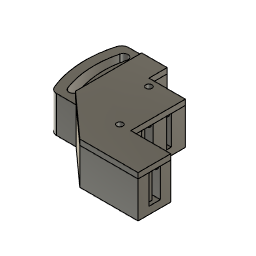
switch_connectors (Autodesk Fusion 360 design; units mm, degrees)
Autodesk Fusion 360 part; units mm, degrees
note: some values were not read from the file. Chosen so that the rebuilt part matches the saved one: which bodies a step acts on; which face or edge a step refers to. Set by a fixed rule: which sketch regions a step uses.
ref_plane "WorkPlane1" through (11.25, 0, 0) normal (1, 0, 0) x (0, 1, 0)
sketch "switch_connector" plane through (0, 0, 0) normal (0, 0, 1) x (1, 0, 0)
  line L0 (-55, 15) -> (-25, 15)
  line L1 (-25, 15) -> (-25, 0)
  line L2 (-25, 0) -> (-55, 0)
  line L3 (-55, 0) -> (-55, 15)
  line L4 (-44, -3) -> (-44, 0)
  line L5 (-43.2133, 0) -> (-43.2133, -4)
  line L6 (-43.2133, -4) -> (-55, -4)
  line L7 (-55, -4) -> (-55, -3)
  line L8 (-55, -3) -> (-44, -3)
  line L9 (-66, 5) -> (-55, 5)
  line L10 (-66, 5) -> (-66, 6)
  line L11 (-66, 6) -> (-55, 6)
  line L12 (-66, 10) -> (-66, 11)
  line L13 (-66, 11) -> (-55, 11)
  line L14 (-55, 10) -> (-66, 10)
  line L15 (-72, 15) -> (-44, 15)
  line L16 (-44, 15) -> (-44, -9)
  line L17 (-44, -9) -> (-72, -9)
  line L18 (-72, -9) -> (-72, 15)
  line L19 (-60, -9) -> (-72, 1.8)
  line L20 (-55, 3.5) -> (-66, 3.5)
  line L21 (-66, 3.5) -> (-66, 3)
  line L22 (-66, 3) -> (-55, 3)
  circle A0 centre (-61, 2.5) radius 1.0194
  line L23 (-63, -1.3962) -> (-60.2264, 1.8361)
  line L24 (-61.8884, 3) -> (-65, 1)
  line L25 (-65, -3) -> (-71, 3)
  line L26 (-71, 3) -> (-71, 15)
  line L27 (-65, 1) -> (-68, 4.3653)
  line L28 (-68, 4.3653) -> (-68, 15)
  line L29 (-56, 3.5) -> (-56, 5)
  line L30 (-44, -5.5) -> (-55, -5.5)
  line L31 (-55, -5.5) -> (-55, -6)
  line L32 (-55, -6) -> (-44, -6)
  line L33 (-44, -6) -> (-44, -5.5)
  line L34 (-45, -5.5) -> (-45, -4)
  circle A1 centre (-55.5, -6.5) radius 1.118
  line L35 (-63, -1.3962) -> (-55, -5.5)
  line L36 (-65, -3) -> (-58.0664, -7.5028)
  line L37 (-58.0664, -7.5028) -> (-55.5506, -7.6169)
  circle A2 centre (-58, 0) radius 0.65
  arc A3 (-75, 18) -> (-74.1574, 3.3947) centre (-52, 12) ccw
  circle A4 centre (-75, 18) radius 1.25
  circle A5 centre (-74.1574, 3.3947) radius 1.25
  line L38 (-74.0903, 17.5501) -> (-74.0625, 17.6607)
  arc A6 (-78.4578, 19.5487) -> (-77.3721, 1.3578) centre (-52, 12) ccw
  line L39 (-71, 15) -> (-71, 19)
  line L40 (-73, 21) -> (-76.5346, 21)
  line L41 (-75.5278, 0.1314) -> (-72, 0.1314)
  arc A7 (-71, 19) -> (-73, 21) centre (-73, 19) ccw
  arc A8 (-76.5346, 21) -> (-78.4578, 19.5487) centre (-76.5346, 19) ccw
  arc A9 (-77.3721, 1.3578) -> (-75.5278, 0.1314) centre (-75.5278, 2.1314) ccw
  arc A10 (-76.2263, 18.2423) -> (-75.3023, 2.896) centre (-52, 12) ccw
  arc A11 (-73.8338, 17.5501) -> (-73.0477, 3.9681) centre (-52, 12) ccw
  line L42 (-72, 12.1082) -> (-65, 12.1082)
  line L43 (-65, 12.1082) -> (-65, 20)
  line L44 (-65, 20) -> (-72, 20)
  line L45 (-72, 20) -> (-72, 12.1082)
  line L46 (-67, 20) -> (-67, 15)
  circle A12 centre (-63, 13) radius 0.65
  line L47 (-72, 0.1314) -> (-70.146, 0.1314)
  dimension "d55" = 30
  dimension "d56" = 15
  dimension "d62" = 1.3
  dimension "d79" = 2.5
  dimension "d80" = 2.5
  dimension "d81" = 2
  dimension "d92" = 1.3
  constraint horizontal L0
  constraint vertical L1
  constraint horizontal L2
  constraint vertical L3
  constraint coincident L2 L4.end
  constraint perpendicular L2 L4
  constraint coincident L2 L5.start
  constraint perpendicular L2 L5
  constraint perpendicular L5 L6
  constraint perpendicular L6 L7
  constraint perpendicular L4 L8
  constraint coincident L3 L9.end
  constraint perpendicular L3 L9
  constraint perpendicular L9 L10
  constraint coincident L3 L11.end
  constraint perpendicular L3 L11
  constraint perpendicular L11 L12
  constraint coincident L3 L13.end
  constraint perpendicular L3 L13
  constraint coincident L3 L14.start
  constraint perpendicular L12 L14
  constraint horizontal L15
  constraint vertical L16
  constraint horizontal L17
  constraint vertical L18
  constraint coincident L17 L19.start
  constraint coincident L18 L19.end
  constraint coincident L3 L20.start
  constraint perpendicular L3 L20
  constraint perpendicular L20 L21
  constraint coincident L3 L22.end
  constraint perpendicular L3 L22
  constraint coincident A0 L23.end
  constraint tangent A0 L23
  constraint coincident A0 L24.start
  constraint coincident L22 L24.start
  constraint coincident L15 L26.end
  constraint perpendicular L15 L26
  constraint coincident L15 L28.end
  constraint perpendicular L15 L28
  constraint coincident L20 L29.start
  constraint coincident L9 L29.end
  constraint perpendicular L9 L29
  constraint horizontal L30
  constraint vertical L31
  constraint horizontal L32
  constraint vertical L33
  constraint coincident L16 L30.start
  constraint coincident L30 L34.start
  constraint coincident L6 L34.end
  constraint perpendicular L6 L34
  constraint coincident L30.end A1
  constraint coincident A1 L37.end
  constraint tangent A1 L37
  constraint coincident A3.start A4.centre
  constraint coincident A3.end A5.centre
  constraint vertical L39
  constraint perpendicular L39 L40
  constraint coincident L18 L41.end
  constraint perpendicular L18 L41
  constraint tangent L40 A7
  constraint tangent L39 A7
  constraint tangent A6 A8
  constraint tangent L40 A8
  constraint equal A7 A8
  constraint tangent L41 A9
  constraint tangent A6 A9
  constraint equal A7 A9
  constraint coincident A4 A10.start
  constraint coincident A3.centre A6.centre
  constraint coincident A4 A11.start
  constraint horizontal L42
  constraint vertical L43
  constraint horizontal L44
  constraint vertical L45
  constraint coincident L18 L42.start
  constraint coincident L44 L46.start
  constraint coincident L15 L46.end
  constraint perpendicular L15 L46
  constraint coincident L19 L47.end
  constraint perpendicular L18 L47
  measures "d55" distance of L0.start L0.end
  measures "d56" distance of L0.start L2.end
  measures "d62" diameter of A2
  measures "d79" diameter of A4
  measures "d80" diameter of A5
  measures "d81" radius of A7
  measures "d92" diameter of A12
extrude "Extrude11" add sketch "switch_connector" along normal blind 10 contours L3 L9 L10 L11 L12 L13 L14 L15 L20 L21 L22 A0 L24 L27 L28 L29 L42 L43 | L15 L28 L42 L43 | L2 L3 L4 L6 L7 L8 L16 L22 A0 L23 L30 L34 L35 | L15 L18 L26 L42 L45 | L16 L17 L18 L19 L25 L26 L32 A1 L36 L37 L42 | L20 L21 L22 A0 | L20 A0 makes body 1 at (-58.6667, 7.3333, 0) makes body 2 at (-64, -5.4, 3.3333) makes body 3 at (-51.3333, -3, 3.3333)
extrude "Extrude12" add sketch "switch_connector" along normal blind 2 contours L3 L9 L10 L11 L12 L13 L14 L15 L20 L21 L22 A0 L24 L27 L28 L29 L42 L43 | L3 L12 L13 L14 | L15 L28 L42 L43 | L2 L3 L4 L6 L7 L8 L16 L22 A0 L23 L30 L34 L35 | L6 L7 L8 L16 | L3 L9 L10 L11 | L15 L26 L28 L42 | A0 L23 L24 L25 L26 L27 L28 A1 L35 L36 L37 L42 | L3 L20 L22 A0 | L6 L16 L30 L34 | L3 L9 L20 L29 | L15 L18 L26 L42 L45 | L16 L17 L18 L19 L25 L26 L32 A1 L36 L37 L42 | L22 A0 | L20 L22 A0 | L16 L30 L32 L33 A1 | L20 L21 L22 A0 | L31 L32 A1 | L31 L32 A1 | A2 | A12 bodies 1 3 2
move_face "OffsetFaces1" offset -0.15 6 faces at (-62.3333, 11, 4.6667) (-62.3333, 6, 4.6667) (-51.3333, -3, 4.6667) (-48.3333, -4, 4.6667) (-62.6667, 5, 4.6667) (-58.6667, 10, 4.6667) on bodies 1
extrude "Extrude13" add sketch "switch_connector" along normal blind 10 and the other way blind -9 separate body contours L15 L26 L28 L42 | A0 L23 L24 L25 L26 L27 L28 A1 L35 L36 L37 L42 | L22 A0 | L20 L22 A0 | L31 L32 A1 picked at (-55.8194, -6.8957) makes body 4
extrude "Extrude14" add sketch "switch_connector" along normal blind 10 and the other way blind -9.5 separate body contours L3 L12 L13 L14 | L6 L7 L8 L16 | L3 L9 L10 L11 | L3 L20 L22 A0 | L20 L22 A0 | L16 L30 L32 L33 A1 | L20 L21 L22 A0 makes body 5 at (-62.3333, 3.1667, 9.5) makes body 6 at (-62.3333, 5.6667, 9.5) makes body 7 at (-47.6667, -3.6667, 9.5) makes body 8 at (-62.3333, 10.6667, 9.5) makes body 9 at (-47.6667, -5.5, 9.6667)
move_face "OffsetFaces2" offset -0.2 15 faces at (-62.3333, 3, 9.6667) (-58.6667, 3.5, 9.6667) (-55, 3.1667, 9.6667) (-62.3333, 5, 9.6667) (-62.3333, 6, 9.6667) (-55, 5.3333, 9.6667) (-58.6667, 10, 9.6667) (-62.3333, 11, 9.6667) (-55, 10.3333, 9.6667) (-51, -6, 9.6667) (-47.6667, -5.5, 9.6667) (-44, -5.6667, 9.6667) (-47.6667, -4, 9.6667) (-51.3333, -3, 9.6667) (-44, -3.3333, 9.6667) on bodies 5 6 7 8 9
move_face "OffsetFaces3" offset -0.2 9 faces at (-71, 13.0721, 9.3333) (-70, 15, 9.3333) (-68, 13.0721, 9.3333) (-66, 2.1218, 9.3333) (-62.9256, 2.3333, 9.3333) (-60.3333, -2.7641, 9.3333) (-62.6888, -4.5009, 9.3333) (-67, -1, 9.3333) (-57.2278, -7.5409, 9.3333) on bodies 4
move_face "OffsetFaces4" offset -0.2 9 faces at (-57.1825, -7.3427, 9.6667) (-54.8497, -7.148, 9.6667) (-54.707, -6.0375, 9.6667) (-62.1647, -0.4228, 9.3333) (-60.0924, 2.0358, 9.6667) (-60.0037, 2.7161, 9.6667) (-60.3631, 3.296, 9.6667) (-60.934, 3.5, 9.3333) (-61.2473, 3.489, 9.6667) on bodies 4
extrude "Extrude15" add sketch "switch_connector" along normal blind 10 and the other way blind -11.5 contours L3 L9 L10 L11 L12 L13 L14 L15 L20 L21 L22 A0 L24 L27 L28 L29 L42 L43 | L3 L12 L13 L14 | L15 L28 L42 L43 | L15 L43 L44 L46 | L2 L3 L4 L6 L7 L8 L16 L22 A0 L23 L30 L34 L35 | L6 L7 L8 L16 | L3 L9 L10 L11 | L15 L26 L28 L42 | A0 L23 L24 L25 L26 L27 L28 A1 L35 L36 L37 L42 | L3 L20 L22 A0 | L6 L16 L30 L34 | L3 L9 L20 L29 | L15 L18 L26 L42 L45 | L15 L39 A7 L44 L45 | L16 L17 L18 L19 L25 L26 L32 A1 L36 L37 L42 | L22 A0 | L20 L22 A0 | L16 L30 L32 L33 A1 | L20 L21 L22 A0 | L20 A0 | L31 L32 A1 | L31 L32 A1 bodies 4 5 6 7 8 9
move_face "OffsetFaces5" offset -0.2 1 faces at (-57.9838, 0.6498, 10.5) on bodies 4
extrude "Extrude16" add sketch "switch_connector" along normal blind 10 contours L15 L43 L44 L46 | L15 L39 A7 L44 L45 | L18 A6 L40 L41 A7 A8 A9 L44 L45 | L18 L19 L47 bodies 1
extrude "Extrude17" add sketch "switch_connector" along normal blind 4 contours L15 L39 A7 L44 L46 bodies 1
extrude "Extrude18" add sketch "switch_connector" along normal blind 11.5 and the other way blind -7 contours L15 L39 A7 L44 L46 bodies 4
extrude "Extrude19" add 1 faces at (-69.9333, 14.8, 9.3333) along direction (0, 1, 0) blind 0.2 on bodies 4 bodies 4
move_face "OffsetFaces6" offset -0.2 1 faces at (-62.4819, 13.3925, 10.5) on bodies 4
mirror "Mirror1" about plane through (0, 0, 0) normal (1, 0, 0) of bodies 1 4 makes body 10 at (63.382, 5.0438, 0) makes body 11 at (64.6305, 4.8167, 11.5)
hidden bodies 10 11
named bodies: "switch_connector", "switch_connector_top", "switch_connector_other", "switch_connector_top_other"
